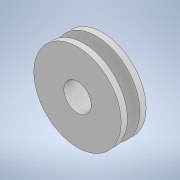
# Autodesk Inventor part: Return_Spool
Saved by Autodesk Inventor 2022 (Build 260153070, 153G)
## iProperties
Created: 2022-03-05
Part Number: Return_Spool
Material: Generic
Document SubType Name: Modeling
Designer: a laptop
Density: 1 g/cm^3
Appearance: Default
Author: a laptop
Autodesk Inventor part; units mm, degrees
ref_plane "YZ Plane" through (0, 0, 0) normal (1, 0, 0) x (0, 1, 0)
ref_plane "XZ Plane" through (0, 0, 0) normal (0, 1, 0) x (-1, 0, 0)
ref_plane "XY Plane" through (0, 0, 0) normal (0, 0, 1) x (1, 0, 0)
sketch "Sketch1" plane through (0, 0, 0) normal (0, 0, 1) x (1, 0, 0)
  circle A0 centre (0, 0) radius 13
  circle A1 centre (0, 0) radius 11
  circle A2 centre (0, 0) radius 35
  dimension "d0" = 26
  dimension "d1" = 22
  dimension "d2" = 70
  constraints: 3 centre point, 3 coincident
  measures "d0" diameter of A0
  measures "d1" diameter of A1
  measures "d2" diameter of A2
extrude "Extrusion1" add sketch "Sketch1" along normal blind 15 and the other way blind 5 contours A0
extrude "Extrusion2" add sketch "Sketch1" along normal blind 15 and the other way blind 5 contours A2
extrude "Extrusion4" cut sketch "Sketch1" along normal blind 10 contours A2
body "Solid1"
